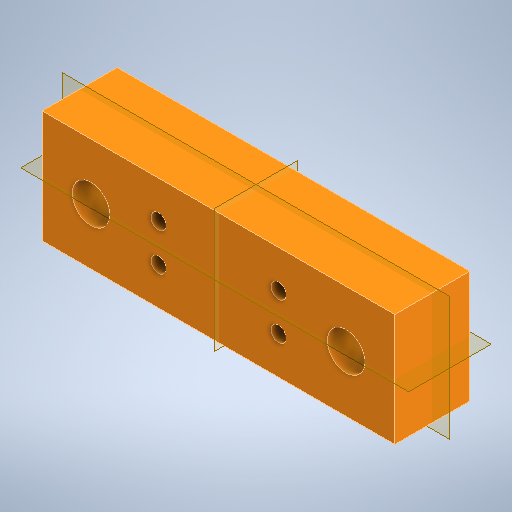
# Autodesk Inventor part: suporte_motor_001
Saved by Autodesk Inventor 2026 (Build 300175000, 175)
## iProperties
Created: 2025-11-26
Part Number: suporte_motor_001
Material: ABS Plastic
Document SubType Name: Modeling
Designer: Carlos Dias
Density: 1.06 g/cm^3
Appearance: Orange
Author: Carlos Dias
Autodesk Inventor part; units mm, degrees
sketch "Sketch1" plane through (0, 0, 0) normal (0, 0, 1) x (1, 0, 0)
  line L0 (-23.5, 7.5) -> (23.5, 7.5)
  line L1 (23.5, 7.5) -> (23.5, -7.5)
  line L2 (23.5, -7.5) -> (-23.5, -7.5)
  line L3 (-23.5, -7.5) -> (-23.5, 7.5)
  line L4 (-23.5, 7.5) -> (23.5, -7.5) construction
  line L5 (23.5, 7.5) -> (-23.5, -7.5) construction
  circle A0 centre (17, 0) radius 2.5
  circle A1 centre (8, 2.5) radius 1
  circle A2 centre (8, -2.5) radius 1
  line L6 (8, 2.5) -> (8, -2.5) construction
  line L7 (0, 7.5) -> (0, -7.5) construction
  circle A3 centre (-17, 0) radius 2.5
  circle A4 centre (-8, 2.5) radius 1
  circle A5 centre (-8, -2.5) radius 1
  point P0 (0, 0)
  point P1 (0, 0)
  point P2 (8, 0)
  point P3 (0, 0)
  dimension "d0" = 47
  dimension "d1" = 15
  dimension "d6" = 5
  dimension "d7" = 17
  dimension "d8" = 2
  dimension "d9" = 2
  dimension "d10" = 8
  dimension "d11" = 5
  constraints: 16 end point, 6 centre point, 6 midpoint, 4 coincident, 3 symmetric about line, 2 horizontal alignment, 2 parallel, 2 vertical, 1 horizontal, 1 perpendicular, 1 vertical alignment, 3 other
  measures "d0" distance of L0.start L0.end
  measures "d1" distance of L0.end L1.end
  measures "d6" diameter of A0
  measures "d7" distance of point (0, 0) A0.centre
  measures "d8" diameter of A1
  measures "d9" diameter of A2
  measures "d10" distance of point (0, 0) point (8, 0)
  measures "d11" distance of L6.start L6.end
extrude "Extrusion1" add sketch "Sketch1" along normal mid plane 10
body "Solid1"
